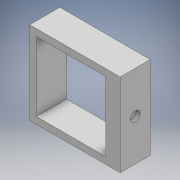
# Autodesk Inventor part: pid-holder
Saved by Autodesk Inventor 2018 (Build 220112000, 112)
## iProperties
Created: 2019-06-13
Part Number: pid-holder
Material: Generic
Document SubType Name: Modeling
Designer: jstklein
Density: 1 g/cm^3
Appearance: Default
Author: jstklein
Autodesk Inventor part; units mm, degrees
ref_plane "YZ Plane" through (0, 0, 0) normal (1, 0, 0) x (0, 1, 0)
ref_plane "XZ Plane" through (0, 0, 0) normal (0, 1, 0) x (-1, 0, 0)
ref_plane "XY Plane" through (0, 0, 0) normal (0, 0, 1) x (1, 0, 0)
sketch "Sketch1" plane through (0, 0, 0) normal (0, 1, 0) x (-1, 0, 0)
  line L0 (23, 23) -> (-23, 23)
  line L1 (-23, 23) -> (-23, -23)
  line L2 (-23, -23) -> (23, -23)
  line L3 (23, -23) -> (23, 23)
  line L4 (23, 23) -> (-23, -23) construction
  line L5 (-23, 23) -> (23, -23) construction
  line L6 (27.5, 27.5) -> (-27.5, 27.5)
  line L7 (-27.5, 27.5) -> (-27.5, -27.5)
  line L8 (-27.5, -27.5) -> (27.5, -27.5)
  line L9 (27.5, -27.5) -> (27.5, 27.5)
  line L10 (27.5, 27.5) -> (-27.5, -27.5) construction
  line L11 (-27.5, 27.5) -> (27.5, -27.5) construction
  line L12 (27.5, 27.5) -> (27.5, -27.5)
  line L13 (27.5, -27.5) -> (-32.5, -27.5)
  line L14 (-32.5, -27.5) -> (-32.5, 27.5)
  line L15 (-32.5, 27.5) -> (27.5, 27.5)
  point P0 (0, 0)
  dimension "d0" = 46
  dimension "d1" = 46
  dimension "d2" = 55
  dimension "d3" = 55
  dimension "d4" = 60
  constraints: 32 end point, 7 equal length, 4 midpoint, 3 perpendicular, 2 horizontal
  measures "d0" distance of L2.end L1.end
  measures "d1" distance of L1.end L0.end
  measures "d2" distance of L8.end L7.end
  measures "d3" distance of L7.end L6.end
  measures "d4" distance of L8.end L13.end
extrude "Extrusion1" add sketch "Sketch1" along normal blind 20
hole "Hole1" at (23, 10, 0) direction (1, 0, 0) diameter 6.45 end through all counterbore diameter 10.525 counterbore depth 6.85
body "Solid1"
